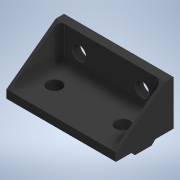
# Autodesk Inventor part: Soporte Cajas
Saved by Autodesk Inventor 2020.3 (Build 243373000, 373)
## iProperties
Created: 2021-03-02
Part Number: Soporte Cajas
Material: Rubber, Silicone
Document SubType Name: Modeling
Designer: juanp
Density: 1.25 g/cm^3
Appearance: Rubber - Black
Author: juanp
Autodesk Inventor part; units mm, degrees
ref_plane "YZ Plane" through (0, 0, 0) normal (1, 0, 0) x (0, 1, 0)
ref_plane "XZ Plane" through (0, 0, 0) normal (0, 1, 0) x (-1, 0, 0)
ref_plane "XY Plane" through (0, 0, 0) normal (0, 0, 1) x (1, 0, 0)
sketch "Sketch1" plane through (0, 0, 0) normal (0, 1, 0) x (-1, 0, 0)
  line L0 (0, 0) -> (-40, 0)
  line L1 (-40, 0) -> (-40, -21)
  line L2 (-40, -21) -> (0, -21)
  line L3 (0, -21) -> (0, 0)
  circle A0 centre (-7.5, -10) radius 2.65
  circle A1 centre (-32.5, -10) radius 2.65
  line L4 (-7.5, -10) -> (-32.5, -10) construction
  line L5 (0, -21) -> (-40, -21)
  line L6 (-40, -21) -> (-40, -18)
  line L7 (-40, -18) -> (0, -18)
  line L8 (0, -18) -> (0, -21)
  line L9 (-40, -21) -> (-39, -21)
  line L10 (-39, -21) -> (-39, 0)
  line L11 (-39, 0) -> (-40, 0)
  line L12 (-40, 0) -> (-40, -21)
  line L13 (0, 0) -> (-1, 0)
  line L14 (-1, 0) -> (-1, -21)
  line L15 (-1, -21) -> (0, -21)
  line L16 (0, -21) -> (0, 0)
  line L17 (-32.5, -10) -> (-40, -10) construction
  line L18 (-7.5, -10) -> (0, -10) construction
  point P0 (-1, -18)
  point P1 (-39, -18)
  dimension "d0" = 40
  dimension "d1" = 21
  dimension "d3" = 5.3
  dimension "d4" = 3
  dimension "d9" = 1
  dimension "d10" = 1
  dimension "d23" = 11
  dimension "d24" = 25
  constraints: 38 end point, 8 parallel, 6 perpendicular, 5 point on line, 4 horizontal, 2 centre point, 2 collinear, 1 equal radius
  measures "d0" distance of L2.end L1.end
  measures "d1" distance of L1.end L0.end
  measures "d3" diameter of A0
  measures "d4" distance between parallel lines of L2 L7
  measures "d9" distance between parallel lines of L3 L14
  measures "d10" distance between parallel lines of L10 L1
  measures "d23" distance between parallel lines of L4 L2
  measures "d24" distance of L4.start L4.end
extrude "Extrusion1" add sketch "Sketch1" along normal blind 3
extrude "Extrusion2" add sketch "Sketch1" along normal blind 16.333 contours L3 L2 L14 L7 | L14 L2 L10 L7 | L10 L2 L1 L7
ref_plane "Work Plane1" through (0, 3, 0) normal (0, 0.8035643, 0.5952179) x (1, 0, 0)
extrude "Extrusion3" add sketch "Sketch1" along normal up to surface contours L3 L7 L14 L0 | L10 L7 L1 L0 surface through (0, 3, 0) normal (0, 0.8035643, 0.5952179)
sketch "Sketch3" plane through (1, 3, -18) normal (0, 0, 1) x (1, 0, 0)
  line L0 (0, 13.333) -> (0, 0) projected
  line L1 (0, 13.333) -> (0, 0) projected
  line L2 (38, 0) -> (0, 0) projected
  line L3 (38, 0) -> (38, 13.333) projected
  line L4 (0, 13.333) -> (38, 13.333) projected
  line L5 (0, 6.6665) -> (7.5, 6.6665) construction
  line L6 (7.5, 6.6665) -> (30.5, 6.6665) construction
  line L7 (30.5, 6.6665) -> (38, 6.6665) construction
  circle A0 centre (7.5, 6.6665) radius 2.65
  circle A1 centre (30.5, 6.6665) radius 2.65
  point P0 (-1, -3)
  dimension "d13" = 7.5
  dimension "d14" = 5.3
  constraints: 6 end point, 2 centre point, 2 coincident, 2 midpoint, 1 collinear, 1 equal radius, 1 horizontal, 1 point on line
  measures "d13" distance of L5.start L5.end
  measures "d14" diameter of A1
extrude "Extrusion4" cut sketch "Sketch3" against normal through all contours A0 | A1
ref_plane "Work Plane2" through (20, 0, -21) normal (-1, 0, 0) x (0, 0, 1)
sketch "Sketch5" plane through (0, 0, 0) normal (0, -1, 0) x (1, 0, 0)
  line L0 (0, -5.625) -> (40, -5.625)
  line L1 (40, -5.625) -> (40, -14.375)
  line L2 (40, -14.375) -> (0, -14.375)
  line L3 (0, -14.375) -> (0, -5.625)
  line L4 (0, -21) -> (0, 0) projected
  line L5 (40, 0) -> (40, -21) projected
  line L6 (0, -10) -> (40, -10) construction
  circle A0 centre (7.5, -10) radius 2.65 projected
  circle A1 centre (32.5, -10) radius 2.65 projected
  dimension "d17" = 8.75
  constraints: 10 end point, 2 collinear, 2 midpoint, 2 parallel, 1 horizontal, 1 perpendicular, 1 point on line
  measures "d17" distance between parallel lines of L0 L2
extrude "Extrusion5" add sketch "Sketch5" along normal blind 1.35
chamfer "Chamfer1" distance 1.35 angle 45 2 edges at (20, -1.35, -5.625) (20, -1.35, -14.375)
fillet "Fillet1" radius 2 5 edges at (1, 3, -9) (1, 9.6665, -18) (20, 3, -18) (39, 9.6665, -18) (39, 3, -9)
body "Solid1"
